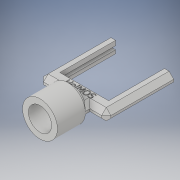
# Autodesk Inventor part: 6 Kamerahaltung
Saved by Autodesk Inventor 2018.3 (Build 223284000, 284)
## iProperties
Created: 2018-11-08
Part Number: 6 Kamerahaltung
Material: Generisch
Document SubType Name: Modeling
Designer: pgmadmin
Density: 1 g/cm^3
Appearance: Vorgabe
Author: pgmadmin
Autodesk Inventor part; units mm, degrees
ref_plane "YZ Plane" through (0, 0, 0) normal (1, 0, 0) x (0, 1, 0)
ref_plane "XZ Plane" through (0, 0, 0) normal (0, 1, 0) x (-1, 0, 0)
ref_plane "XY Plane" through (0, 0, 0) normal (0, 0, 1) x (1, 0, 0)
sketch "Skizze1" plane through (0, 0, 0) normal (0, 0, 1) x (1, 0, 0)
  line L0 (0, 0) -> (25, 0)
  line L1 (25, 0) -> (25, 24)
  line L2 (0, 24) -> (0, 0)
  line L3 (0, 24) -> (-5, 24)
  line L4 (-5, 24) -> (-5, -5)
  line L5 (-5, -5) -> (30, -5)
  line L6 (30, -5) -> (30, 24)
  line L7 (30, 24) -> (25, 24)
  constraints: 16 end point, 5 perpendicular, 2 horizontal, 1 parallel, 1 point on line
extrude "Extrusion1" add sketch "Skizze1" along normal blind 12
sketch "Skizze2" plane through (0, 0, 0) normal (0, 0, -1) x (-1, 0, 0)
  line L0 (-25, 24) -> (-23, 24)
  line L1 (-23, 24) -> (-23, -1.0226)
  line L2 (-23, -1.0226) -> (-25, -1.0226)
  line L3 (-25, -1.0226) -> (-25, 24)
  line L4 (0, 0) -> (0, 24) projected
  line L5 (0, 24) -> (-2, 24)
  line L6 (-2, 24) -> (-2, -3.2856)
  line L7 (-2, -3.2856) -> (0, -3.2856)
  line L8 (0, -3.2856) -> (0, 24)
  dimension "d7" = 2
  dimension "d8" = 2
  constraints: 16 end point, 4 parallel, 2 horizontal, 2 perpendicular
  measures "d7" distance of L1.end L2.end
  measures "d8" distance of L7.end L6.end
extrude "Extrusion2" add sketch "Skizze2" against normal blind 3
sketch "Skizze3" plane through (0, 0, 12) normal (0, 0, 1) x (1, 0, 0)
  line L0 (0, 24) -> (-5, 24) projected
  line L1 (0, 24) -> (2, 24)
  line L2 (2, 24) -> (2, -1.1552)
  line L3 (2, -1.1552) -> (0, -1.1552)
  line L4 (0, -1.1552) -> (0, 24)
  line L5 (25, 24) -> (23, 24)
  line L6 (23, 24) -> (23, -1.1552)
  line L7 (23, -1.1552) -> (25, -1.1552)
  line L8 (25, -1.1552) -> (25, 24)
  point P0 (0, 0)
  constraints: 16 end point, 4 parallel, 2 horizontal, 2 perpendicular, 1 point on line
extrude "Extrusion3" add sketch "Skizze3" against normal blind 8
sketch "Skizze4" plane through (-5, 24, 12) normal (0, 1, 0) x (1, 0, 0)
  line L0 (7, 12) -> (7, 9) projected
  line L1 (3, 11) -> (3, 6)
  line L2 (3, 6) -> (32, 6)
  line L3 (7, 8) -> (7, 0) projected
  line L4 (32, 6) -> (32, 11)
  line L5 (5, 9) -> (5, 8) projected
  line L6 (30, 9) -> (30, 8) projected
  line L7 (5, 8) -> (7, 8) projected
  line L8 (3, 11) -> (32, 11)
  line L9 (7, 9) -> (5, 9) projected
  line L10 (0, 12) -> (0, 0) projected
  line L11 (35, 0) -> (28, 0) projected
  line L12 (0, 12) -> (35, 12)
  line L13 (35, 12) -> (35, 0)
  line L14 (35, 0) -> (0, 0)
  line L15 (0, 0) -> (0, 12)
  point P0 (5, 12)
  dimension "d16" = 2
  constraints: 16 end point, 3 perpendicular, 2 horizontal, 2 parallel
  measures "d16" distance between parallel lines of L8 L9
extrude "Extrusion4" cut sketch "Skizze4" against normal blind 90.5 contours L12 L13 L11 L14 L3 L2 L4 L8 L0 | L0 L8 L1 L2 L3 L14 L10 L12
sketch "Skizze5" plane through (23, 24, 3) normal (0, 1, 0) x (1, 0, 0)
  line L0 (2.5, -1) -> (-23.5, -1)
  line L1 (-23.5, -1) -> (-23.5, 0.5)
  line L2 (-23.5, 0.5) -> (2.5, 0.5)
  line L3 (2.5, 0.5) -> (2.5, -1)
  line L4 (2, 0) -> (2, -1) projected
  line L5 (-23, 0) -> (-23, -1) projected
  point P0 (-23, 3)
  dimension "d19" = 26
  dimension "d20" = 1.5
  dimension "d21" = 0.5
  dimension "d22" = 0.5
  constraints: 8 end point, 2 parallel, 1 horizontal, 1 perpendicular
  measures "d19" distance of L1.end L2.end
  measures "d20" distance of L0.end L1.end
  measures "d21" distance between parallel lines of L4 L3
  measures "d22" distance between parallel lines of L1 L5
extrude "Extrusion5" cut sketch "Skizze5" against normal blind 24
sketch "Skizze6" plane through (-2, -5, 6) normal (0, -1, 0) x (1, 0, 0)
  circle A0 centre (14.5, -2.5) radius 7.5
  line L0 (29, 0) -> (0, 0) projected
  point P0 (2, -6)
  dimension "d25" = 15
  dimension "d26" = 2.5
  constraints: 1 centre point
  measures "d25" diameter of A0
  measures "d26" distance from line of L0 A0.centre
extrude "Extrusion6" add sketch "Skizze6" along normal blind 14
chamfer "Fase2" distance 2 angle 45 2 edges at (12.5, -5, 11) (12.5, -5, -4)
chamfer "Fase3" distance 2 angle 45 12 edges at (-2, 9.5, 1) (-2, 9.5, 6) (27, 9.5, 6) (23.2855, -5, 6) (1.7145, -5, 6) (5.4289, -6, 6) (19.5711, -6, 6) (5.4289, -6, 1) (19.5711, -6, 1) (27, 9.5, 1) (27, -5, 3.5) (-2, -5, 3.5)
chamfer "Fase4" distance 2 angle 45 4 edges at (22.2855, -5, 1) (18.5711, -5, 1) (6.4289, -5, 1) (2.7145, -5, 1)
sketch "Skizze7" plane through (12.5, -19, 3.5) normal (0, -1, 0) x (1, 0, 0)
  circle A0 centre (0, 0) radius 5
  point P0 (-12.5, -3.5)
  dimension "d42" = 10
  constraints: 1 centre point
  measures "d42" diameter of A0
extrude "Extrusion7" cut sketch "Skizze7" against normal blind 10
sketch "Skizze8" plane through (2, 0, 6) normal (0, 0, 1) x (1, 0, 0)
  line L0 (0, 24) -> (0, 0) projected
  line L1 (0, 24) -> (0, -5)
  line L2 (3.0167, -5) -> (-2, -5) projected
  line L3 (21, 0) -> (21, 24) projected
  line L4 (21, 24) -> (21, -5)
  line L5 (23, -5) -> (17.9833, -5) projected
  line L6 (23, -3) -> (15.5711, -3) projected
  line L7 (21, -3) -> (0, -3)
  line L8 (6.4653, -3) -> (6.1277, -3)
  line L9 (6.1277, -3) -> (6.1277, -1.7568)
  line L10 (6.1277, -1.7568) -> (4.9586, -1.7568)
  line L11 (4.9586, -1.7568) -> (4.9586, -3)
  line L12 (4.9586, -3) -> (4.621, -3)
  line L13 (4.621, -3) -> (4.621, -0.46)
  line L14 (4.621, -0.46) -> (4.9586, -0.46)
  line L15 (4.9586, -0.46) -> (4.9586, -1.4562)
  line L16 (4.9586, -1.4562) -> (6.1277, -1.4562)
  line L17 (6.1277, -1.4562) -> (6.1277, -0.46)
  line L18 (6.1277, -0.46) -> (6.4653, -0.46)
  line L19 (6.4653, -0.46) -> (6.4653, -3)
  spline S0 degree 2 poles (8.5216, -2.047) (8.5216, -2.5286) (8.0584, -3.0535) (7.6715, -3.0535) knots 0 0 0 1 2 2 2
  spline S1 degree 2 poles (7.6715, -3.0535) (7.2742, -3.0535) (6.8193, -2.5122) (6.8193, -2.047) knots 0 0 0 1 2 2 2
  spline S2 degree 2 poles (6.8193, -2.047) (6.8193, -1.5694) (7.2886, -1.0405) (7.6715, -1.0405) knots 0 0 0 1 2 2 2
  spline S3 degree 2 poles (7.6715, -1.0405) (8.0584, -1.0405) (8.5216, -1.5674) (8.5216, -2.047) knots 0 0 0 1 2 2 2
  spline S4 degree 2 poles (8.1902, -2.047) (8.1902, -1.6765) (7.9205, -1.3163) (7.6715, -1.3163) knots 0 0 0 1 2 2 2
  spline S5 degree 2 poles (7.6715, -1.3163) (7.4224, -1.3163) (7.1507, -1.6765) (7.1507, -2.047) knots 0 0 0 1 2 2 2
  spline S6 degree 2 poles (7.1507, -2.047) (7.1507, -2.4072) (7.4224, -2.7777) (7.6715, -2.7777) knots 0 0 0 1 2 2 2
  spline S7 degree 2 poles (7.6715, -2.7777) (7.9185, -2.7777) (8.1902, -2.4134) (8.1902, -2.047) knots 0 0 0 1 2 2 2
  line L20 (9.1782, -3) -> (8.8571, -3)
  line L21 (8.8571, -3) -> (8.8571, -0.3468)
  line L22 (8.8571, -0.3468) -> (9.1782, -0.3468)
  line L23 (9.1782, -0.3468) -> (9.1782, -3)
  line L24 (11.852, -3) -> (11.5144, -3)
  line L25 (11.5144, -3) -> (11.5144, -0.812)
  line L26 (11.5144, -0.812) -> (10.8516, -2.3002)
  line L27 (10.8516, -2.3002) -> (10.6458, -2.3002)
  line L28 (10.6458, -2.3002) -> (9.9892, -0.812)
  line L29 (9.9892, -0.812) -> (9.9892, -3)
  line L30 (9.9892, -3) -> (9.6742, -3)
  line L31 (9.6742, -3) -> (9.6742, -0.46)
  line L32 (9.6742, -0.46) -> (10.1353, -0.46)
  line L33 (10.1353, -0.46) -> (10.7693, -1.8741)
  line L34 (10.7693, -1.8741) -> (11.3827, -0.46)
  line L35 (11.3827, -0.46) -> (11.852, -0.46)
  line L36 (11.852, -0.46) -> (11.852, -3)
  spline S8 degree 2 poles (14.1635, -0.7502) (14.3076, -0.919) (14.4681, -1.413) (14.4681, -1.73) knots 0 0 0 1 2 2 2
  spline S9 degree 2 poles (14.4681, -1.73) (14.4681, -2.0388) (14.3117, -2.5389) (14.1635, -2.7077) knots 0 0 0 1 2 2 2
  spline S10 degree 2 poles (14.1635, -2.7077) (14.0071, -2.8847) (13.5933, -3.0535) (13.3443, -3.0535) knots 0 0 0 1 2 2 2
  spline S11 degree 2 poles (13.3443, -3.0535) (13.087, -3.0535) (12.6753, -2.8786) (12.525, -2.7077) knots 0 0 0 1 2 2 2
  spline S12 degree 2 poles (12.525, -2.7077) (12.3789, -2.5389) (12.2225, -2.0429) (12.2225, -1.73) knots 0 0 0 1 2 2 2
  spline S13 degree 2 poles (12.2225, -1.73) (12.2225, -1.411) (12.381, -0.9252) (12.5271, -0.7502) knots 0 0 0 1 2 2 2
  spline S14 degree 2 poles (12.5271, -0.7502) (12.6753, -0.5814) (13.089, -0.4065) (13.3443, -0.4065) knots 0 0 0 1 2 2 2
  spline S15 degree 2 poles (13.3443, -0.4065) (13.6036, -0.4065) (14.0194, -0.5876) (14.1635, -0.7502) knots 0 0 0 1 2 2 2
  spline S16 degree 2 poles (14.1161, -1.73) (14.1161, -1.4789) (14.0071, -1.0899) (13.9082, -0.9622) knots 0 0 0 1 2 2 2
  spline S17 degree 2 poles (13.9082, -0.9622) (13.8074, -0.8305) (13.5233, -0.6988) (13.3463, -0.6988) knots 0 0 0 1 2 2 2
  spline S18 degree 2 poles (13.3463, -0.6988) (13.1631, -0.6988) (12.8873, -0.8264) (12.7823, -0.9622) knots 0 0 0 1 2 2 2
  spline S19 degree 2 poles (12.7823, -0.9622) (12.6815, -1.0919) (12.5744, -1.483) (12.5744, -1.73) knots 0 0 0 1 2 2 2
  spline S20 degree 2 poles (12.5744, -1.73) (12.5744, -2.2302) (12.9943, -2.7612) (13.3463, -2.7612) knots 0 0 0 1 2 2 2
  spline S21 degree 2 poles (13.3463, -2.7612) (13.6983, -2.7612) (14.1161, -2.2302) (14.1161, -1.73) knots 0 0 0 1 2 2 2
  spline S22 degree 2 poles (15.5467, -3.0453) (15.2709, -3.0453) (14.8839, -2.93) (14.7131, -2.8477) knots 0 0 0 1 2 2 2
  line L37 (14.7131, -2.8477) -> (14.7131, -2.4237)
  line L38 (14.7131, -2.4237) -> (14.7378, -2.4237)
  spline S23 degree 2 poles (14.7378, -2.4237) (14.9045, -2.5801) (15.3265, -2.753) (15.522, -2.753) knots 0 0 0 1 2 2 2
  spline S24 degree 2 poles (15.522, -2.753) (15.8019, -2.753) (16.088, -2.5204) (16.088, -2.329) knots 0 0 0 1 2 2 2
  spline S25 degree 2 poles (16.088, -2.329) (16.088, -2.1767) (15.9378, -1.9873) (15.7752, -1.94) knots 0 0 0 1 2 2 2
  spline S26 degree 2 poles (15.7752, -1.94) (15.6578, -1.907) (15.4623, -1.8617) (15.3162, -1.8247) knots 0 0 0 1 2 2 2
  spline S27 degree 2 poles (15.3162, -1.8247) (15.1844, -1.7897) (14.9765, -1.6847) (14.8963, -1.6003) knots 0 0 0 1 2 2 2
  spline S28 degree 2 poles (14.8963, -1.6003) (14.818, -1.5159) (14.7316, -1.2895) (14.7316, -1.1413) knots 0 0 0 1 2 2 2
  spline S29 degree 2 poles (14.7316, -1.1413) (14.7316, -0.8326) (15.2132, -0.4147) (15.5858, -0.4147) knots 0 0 0 1 2 2 2
  spline S30 degree 2 poles (15.5858, -0.4147) (15.7999, -0.4147) (16.1786, -0.4991) (16.3412, -0.5794) knots 0 0 0 1 2 2 2
  line L39 (16.3412, -0.5794) -> (16.3412, -0.9828)
  line L40 (16.3412, -0.9828) -> (16.3165, -0.9828)
  spline S31 degree 2 poles (16.3165, -0.9828) (16.1951, -0.8717) (15.8163, -0.707) (15.6084, -0.707) knots 0 0 0 1 2 2 2
  spline S32 degree 2 poles (15.6084, -0.707) (15.3738, -0.707) (15.0836, -0.9272) (15.0836, -1.1063) knots 0 0 0 1 2 2 2
  spline S33 degree 2 poles (15.0836, -1.1063) (15.0836, -1.2669) (15.2544, -1.4583) (15.415, -1.5015) knots 0 0 0 1 2 2 2
  spline S34 degree 2 poles (15.415, -1.5015) (15.522, -1.5303) (15.8328, -1.6044) (15.9357, -1.6353) knots 0 0 0 1 2 2 2
  spline S35 degree 2 poles (15.9357, -1.6353) (16.1971, -1.7156) (16.44, -2.0388) (16.44, -2.2755) knots 0 0 0 1 2 2 2
  spline S36 degree 2 poles (16.44, -2.2755) (16.44, -2.4257) (16.3186, -2.7139) (16.2095, -2.8147) knots 0 0 0 1 2 2 2
  spline S37 degree 2 poles (16.2095, -2.8147) (16.088, -2.9259) (15.7793, -3.0453) (15.5467, -3.0453) knots 0 0 0 1 2 2 2
  point P0 (-2, 0)
  constraints: 6 end point, 5 point on line, 2 vertical, 1 horizontal, 1 perpendicular
extrude "Extrusion8" cut sketch "Skizze8" against normal blind 1 contours S37 S22 L7 L6 | L6 L7 S22 L37 L38 S23 S24 S25 S26 S27 S28 S29 S30 L39 L40 S31 S32 S33 S34 S35 S36 S37 | L7 L25 L26 L27 L28 L29 L31 L32 L33 L34 L35 L36 | L7 L21 L22 L23 | L7 L9 L10 L11 L13 L14 L15 L16 L17 L18 L19 | S10 S11 L7 | L7 S11 S12 S13 S14 S15 S8 S9 S10 | S0 S1 L7 | L7 S1 S2 S3 S0
sketch "Skizze9" plane through (23, 0, 1) normal (0, 0, -1) x (-1, 0, 0)
  line L0 (0, 0) -> (0, 24) projected
  line L1 (0, 24) -> (0, -4.7514)
  line L2 (21, 24) -> (23, 24) projected
  line L3 (21, 24) -> (21, -5.0123)
  line L4 (5.4289, -3) -> (-2, -3) projected
  line L5 (0, -3) -> (21, -3)
  line L6 (16.379, -3) -> (23, -3) projected
  line L7 (6.4653, -3) -> (6.1277, -3)
  line L8 (6.1277, -3) -> (6.1277, -1.7568)
  line L9 (6.1277, -1.7568) -> (4.9586, -1.7568)
  line L10 (4.9586, -1.7568) -> (4.9586, -3)
  line L11 (4.9586, -3) -> (4.621, -3)
  line L12 (4.621, -3) -> (4.621, -0.46)
  line L13 (4.621, -0.46) -> (4.9586, -0.46)
  line L14 (4.9586, -0.46) -> (4.9586, -1.4562)
  line L15 (4.9586, -1.4562) -> (6.1277, -1.4562)
  line L16 (6.1277, -1.4562) -> (6.1277, -0.46)
  line L17 (6.1277, -0.46) -> (6.4653, -0.46)
  line L18 (6.4653, -0.46) -> (6.4653, -3)
  spline S0 degree 2 poles (8.5216, -2.047) (8.5216, -2.5286) (8.0584, -3.0535) (7.6715, -3.0535) knots 0 0 0 1 2 2 2
  spline S1 degree 2 poles (7.6715, -3.0535) (7.2742, -3.0535) (6.8193, -2.5122) (6.8193, -2.047) knots 0 0 0 1 2 2 2
  spline S2 degree 2 poles (6.8193, -2.047) (6.8193, -1.5694) (7.2886, -1.0405) (7.6715, -1.0405) knots 0 0 0 1 2 2 2
  spline S3 degree 2 poles (7.6715, -1.0405) (8.0584, -1.0405) (8.5216, -1.5674) (8.5216, -2.047) knots 0 0 0 1 2 2 2
  spline S4 degree 2 poles (8.1902, -2.047) (8.1902, -1.6765) (7.9205, -1.3163) (7.6715, -1.3163) knots 0 0 0 1 2 2 2
  spline S5 degree 2 poles (7.6715, -1.3163) (7.4224, -1.3163) (7.1507, -1.6765) (7.1507, -2.047) knots 0 0 0 1 2 2 2
  spline S6 degree 2 poles (7.1507, -2.047) (7.1507, -2.4072) (7.4224, -2.7777) (7.6715, -2.7777) knots 0 0 0 1 2 2 2
  spline S7 degree 2 poles (7.6715, -2.7777) (7.9185, -2.7777) (8.1902, -2.4134) (8.1902, -2.047) knots 0 0 0 1 2 2 2
  line L19 (9.1782, -3) -> (8.8571, -3)
  line L20 (8.8571, -3) -> (8.8571, -0.3468)
  line L21 (8.8571, -0.3468) -> (9.1782, -0.3468)
  line L22 (9.1782, -0.3468) -> (9.1782, -3)
  line L23 (11.852, -3) -> (11.5144, -3)
  line L24 (11.5144, -3) -> (11.5144, -0.812)
  line L25 (11.5144, -0.812) -> (10.8516, -2.3002)
  line L26 (10.8516, -2.3002) -> (10.6458, -2.3002)
  line L27 (10.6458, -2.3002) -> (9.9892, -0.812)
  line L28 (9.9892, -0.812) -> (9.9892, -3)
  line L29 (9.9892, -3) -> (9.6742, -3)
  line L30 (9.6742, -3) -> (9.6742, -0.46)
  line L31 (9.6742, -0.46) -> (10.1353, -0.46)
  line L32 (10.1353, -0.46) -> (10.7693, -1.8741)
  line L33 (10.7693, -1.8741) -> (11.3827, -0.46)
  line L34 (11.3827, -0.46) -> (11.852, -0.46)
  line L35 (11.852, -0.46) -> (11.852, -3)
  spline S8 degree 2 poles (14.1635, -0.7502) (14.3076, -0.919) (14.4681, -1.413) (14.4681, -1.73) knots 0 0 0 1 2 2 2
  spline S9 degree 2 poles (14.4681, -1.73) (14.4681, -2.0388) (14.3117, -2.5389) (14.1635, -2.7077) knots 0 0 0 1 2 2 2
  spline S10 degree 2 poles (14.1635, -2.7077) (14.0071, -2.8847) (13.5933, -3.0535) (13.3443, -3.0535) knots 0 0 0 1 2 2 2
  spline S11 degree 2 poles (13.3443, -3.0535) (13.087, -3.0535) (12.6753, -2.8786) (12.525, -2.7077) knots 0 0 0 1 2 2 2
  spline S12 degree 2 poles (12.525, -2.7077) (12.3789, -2.5389) (12.2225, -2.0429) (12.2225, -1.73) knots 0 0 0 1 2 2 2
  spline S13 degree 2 poles (12.2225, -1.73) (12.2225, -1.411) (12.381, -0.9252) (12.5271, -0.7502) knots 0 0 0 1 2 2 2
  spline S14 degree 2 poles (12.5271, -0.7502) (12.6753, -0.5814) (13.089, -0.4065) (13.3443, -0.4065) knots 0 0 0 1 2 2 2
  spline S15 degree 2 poles (13.3443, -0.4065) (13.6036, -0.4065) (14.0194, -0.5876) (14.1635, -0.7502) knots 0 0 0 1 2 2 2
  spline S16 degree 2 poles (14.1161, -1.73) (14.1161, -1.4789) (14.0071, -1.0899) (13.9082, -0.9622) knots 0 0 0 1 2 2 2
  spline S17 degree 2 poles (13.9082, -0.9622) (13.8074, -0.8305) (13.5233, -0.6988) (13.3463, -0.6988) knots 0 0 0 1 2 2 2
  spline S18 degree 2 poles (13.3463, -0.6988) (13.1631, -0.6988) (12.8873, -0.8264) (12.7823, -0.9622) knots 0 0 0 1 2 2 2
  spline S19 degree 2 poles (12.7823, -0.9622) (12.6815, -1.0919) (12.5744, -1.483) (12.5744, -1.73) knots 0 0 0 1 2 2 2
  spline S20 degree 2 poles (12.5744, -1.73) (12.5744, -2.2302) (12.9943, -2.7612) (13.3463, -2.7612) knots 0 0 0 1 2 2 2
  spline S21 degree 2 poles (13.3463, -2.7612) (13.6983, -2.7612) (14.1161, -2.2302) (14.1161, -1.73) knots 0 0 0 1 2 2 2
  spline S22 degree 2 poles (15.5467, -3.0453) (15.2709, -3.0453) (14.8839, -2.93) (14.7131, -2.8477) knots 0 0 0 1 2 2 2
  line L36 (14.7131, -2.8477) -> (14.7131, -2.4237)
  line L37 (14.7131, -2.4237) -> (14.7378, -2.4237)
  spline S23 degree 2 poles (14.7378, -2.4237) (14.9045, -2.5801) (15.3265, -2.753) (15.522, -2.753) knots 0 0 0 1 2 2 2
  spline S24 degree 2 poles (15.522, -2.753) (15.8019, -2.753) (16.088, -2.5204) (16.088, -2.329) knots 0 0 0 1 2 2 2
  spline S25 degree 2 poles (16.088, -2.329) (16.088, -2.1767) (15.9378, -1.9873) (15.7752, -1.94) knots 0 0 0 1 2 2 2
  spline S26 degree 2 poles (15.7752, -1.94) (15.6578, -1.907) (15.4623, -1.8617) (15.3162, -1.8247) knots 0 0 0 1 2 2 2
  spline S27 degree 2 poles (15.3162, -1.8247) (15.1844, -1.7897) (14.9765, -1.6847) (14.8963, -1.6003) knots 0 0 0 1 2 2 2
  spline S28 degree 2 poles (14.8963, -1.6003) (14.818, -1.5159) (14.7316, -1.2895) (14.7316, -1.1413) knots 0 0 0 1 2 2 2
  spline S29 degree 2 poles (14.7316, -1.1413) (14.7316, -0.8326) (15.2132, -0.4147) (15.5858, -0.4147) knots 0 0 0 1 2 2 2
  spline S30 degree 2 poles (15.5858, -0.4147) (15.7999, -0.4147) (16.1786, -0.4991) (16.3412, -0.5794) knots 0 0 0 1 2 2 2
  line L38 (16.3412, -0.5794) -> (16.3412, -0.9828)
  line L39 (16.3412, -0.9828) -> (16.3165, -0.9828)
  spline S31 degree 2 poles (16.3165, -0.9828) (16.1951, -0.8717) (15.8163, -0.707) (15.6084, -0.707) knots 0 0 0 1 2 2 2
  spline S32 degree 2 poles (15.6084, -0.707) (15.3738, -0.707) (15.0836, -0.9272) (15.0836, -1.1063) knots 0 0 0 1 2 2 2
  spline S33 degree 2 poles (15.0836, -1.1063) (15.0836, -1.2669) (15.2544, -1.4583) (15.415, -1.5015) knots 0 0 0 1 2 2 2
  spline S34 degree 2 poles (15.415, -1.5015) (15.522, -1.5303) (15.8328, -1.6044) (15.9357, -1.6353) knots 0 0 0 1 2 2 2
  spline S35 degree 2 poles (15.9357, -1.6353) (16.1971, -1.7156) (16.44, -2.0388) (16.44, -2.2755) knots 0 0 0 1 2 2 2
  spline S36 degree 2 poles (16.44, -2.2755) (16.44, -2.4257) (16.3186, -2.7139) (16.2095, -2.8147) knots 0 0 0 1 2 2 2
  spline S37 degree 2 poles (16.2095, -2.8147) (16.088, -2.9259) (15.7793, -3.0453) (15.5467, -3.0453) knots 0 0 0 1 2 2 2
  point P0 (23, 0)
  constraints: 6 end point, 4 point on line, 1 collinear, 1 horizontal, 1 vertical
extrude "Extrusion9" cut sketch "Skizze9" against normal blind 1 contours L4 L12 L13 L14 L15 L16 L17 L18 L5 L8 L9 L10 | L20 L21 L22 L5 | L30 L31 L32 L33 L34 L35 L5 L24 L25 L26 L27 L28 | S1 S2 S3 S0 L5 | L5 S0 S1 | S11 S12 S13 S14 S15 S8 S9 S10 L5 | L5 S10 S11 | S22 L36 L37 S23 S24 S25 S26 S27 S28 S29 S30 L38 L39 S31 S32 S33 S34 S35 S36 S37 L5 | L5 S37 S22
sketch "Skizze10" plane through (2, 0, 1) normal (0, 1, 0) x (1, 0, 0)
  line L0 (-2, 0) -> (5.1075, 0) projected
  line L1 (21, -1.5) -> (21, 0) projected
  line L2 (0.0059, 0) -> (21, 0)
  line L3 (21, 0) -> (21, -1.5)
  line L4 (21, -1.5) -> (0.0059, -1.5)
  line L5 (0.0059, -1.5) -> (0.0059, 0)
  point P0 (-2, 1)
  constraints: 8 end point, 2 parallel, 1 horizontal, 1 perpendicular, 1 point on line
extrude "Extrusion10" cut sketch "Skizze10" against normal blind 5
